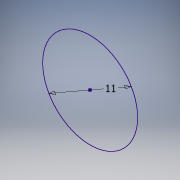
# Autodesk Inventor part: Upper Pneumatic Support
Saved by Autodesk Inventor 2019.4 (Build 234330000, 330)
## iProperties
Created: 2020-01-26
Part Number: Upper Pneumatic Support
Material: Aluminum 6061
Document SubType Name: Modeling
Designer: Mark
Mass: 36.7998 g
Surface Area: 66.9175 cm^2
Volume: 13.6295 cm^3
Density: 2.7 g/cm^3
Appearance: Aluminum - Flat
Author: Mark
Autodesk Inventor part; units mm, degrees
ref_plane "YZ Plane" through (0, 0, 0) normal (1, 0, 0) x (0, 1, 0)
ref_plane "XZ Plane" through (0, 0, 0) normal (0, 1, 0) x (-1, 0, 0)
ref_plane "XY Plane" through (0, 0, 0) normal (0, 0, 1) x (1, 0, 0)
sketch "Sketch1" plane through (0, 0, 0) normal (0, 0, 1) x (1, 0, 0)
  circle A0 centre (0, 0) radius 5.25
  line L0 (-22.5, -22.5) -> (22.5, -22.5)
  line L1 (22.5, -22.5) -> (22.5, 22.5)
  line L2 (22.5, 22.5) -> (-22.5, 22.5)
  line L3 (-22.5, 22.5) -> (-22.5, -22.5)
  line L4 (-22.5, -22.5) -> (22.5, 22.5) construction
  line L5 (22.5, -22.5) -> (-22.5, 22.5) construction
  line L6 (-22.5, 22.5) -> (22.5, 22.5)
  line L7 (22.5, 22.5) -> (22.5, 40)
  line L8 (22.5, 40) -> (-22.5, 40)
  line L9 (-22.5, 40) -> (-22.5, 22.5)
  dimension "d0" = 10.5
  dimension "d1" = 45
  dimension "d2" = 45
  dimension "d3" = 45
  dimension "d4" = 17.5
  constraints: 20 end point, 4 parallel, 2 horizontal, 2 midpoint, 2 perpendicular, 1 centre point, 1 coincident
  measures "d0" diameter of A0
  measures "d1" distance of L2.end L1.end
  measures "d2" distance of L1.end L0.end
  measures "d3" distance of L8.end L7.end
  measures "d4" distance of L7.end L6.end
extrude "Extrusion1" add sketch "Sketch1" along normal blind 5
sketch "Sketch2" plane through (0, 0, 5) normal (0, 0, 1) x (1, 0, 0)
  line L0 (-22.5, 40) -> (-22.5, -22.5) projected
  line L1 (-22.5, 40) -> (22.5, 40)
  line L2 (22.5, 40) -> (22.5, 35)
  line L3 (22.5, 35) -> (-22.5, 35)
  line L4 (-22.5, 35) -> (-22.5, 40)
  point P0 (0, 0)
  dimension "d7" = 45
  dimension "d8" = 5
  constraints: 8 end point, 2 parallel, 1 horizontal, 1 perpendicular
  measures "d7" distance of L2.end L3.end
  measures "d8" distance of L1.end L2.end
extrude "Extrusion2" add sketch "Sketch2" against normal blind 55
sketch "Sketch3" plane through (-22.5, 35, 0) normal (0, -1, 0) x (1, 0, 0)
  line L0 (22.5, -8.25) -> (37.5, -8.25) construction
  line L1 (22.5, -11) -> (37.5, -11)
  line L2 (37.5, -5.5) -> (22.5, -5.5)
  arc A0 (22.5, -5.5) -> (22.5, -11) centre (22.5, -8.25) ccw
  arc A1 (37.5, -11) -> (37.5, -5.5) centre (37.5, -8.25) ccw
  line L3 (22.5, -23.75) -> (37.5, -23.75) construction
  line L4 (22.5, -26.5) -> (37.5, -26.5)
  line L5 (37.5, -21) -> (22.5, -21)
  arc A2 (22.5, -21) -> (22.5, -26.5) centre (22.5, -23.75) ccw
  arc A3 (37.5, -26.5) -> (37.5, -21) centre (37.5, -23.75) ccw
  line L6 (22.5, -23.75) -> (37.5, -23.75) construction
  line L7 (22.5, -39.25) -> (37.5, -39.25) construction
  line L8 (22.5, -42) -> (37.5, -42)
  line L9 (37.5, -36.5) -> (22.5, -36.5)
  arc A4 (22.5, -36.5) -> (22.5, -42) centre (22.5, -39.25) ccw
  arc A5 (37.5, -42) -> (37.5, -36.5) centre (37.5, -39.25) ccw
  line L10 (22.5, -39.25) -> (37.5, -39.25) construction
  line L11 (0, 0) -> (0, -50) projected
  line L12 (45, -50) -> (0, -50) projected
  point P0 (22.5, 0)
  point P1 (30, -8.25)
  point P2 (30, -23.75)
  point P3 (30, -39.25)
  dimension "d11" = 15
  dimension "d12" = 5.5
  dimension "d13" = 15
  dimension "d14" = 0
  dimension "d15" = 5.5
  dimension "d16" = 15
  dimension "d17" = 0
  dimension "d18" = 5.5
  dimension "d19" = 10
  dimension "d20" = 10
  dimension "d21" = 22.5
  dimension "d22" = 22.5
  dimension "d23" = 22.5
  dimension "d24" = 8
  constraints: 28 end point, 12 point on circle, 12 tangent, 6 centre point, 5 parallel, 3 horizontal, 3 midpoint, 2 collinear
  measures "d11" distance of L0.start L0.end
  measures "d12" diameter of A1
  measures "d13" distance of L3.start L3.end
  measures "d14" distance between parallel lines of L3 L6
  measures "d15" diameter of A3
  measures "d16" distance of L7.start L7.end
  measures "d17" distance between parallel lines of L7 L10
  measures "d18" diameter of A5
  measures "d19" distance between parallel lines of L5 L1
  measures "d20" distance between parallel lines of L4 L9
  measures "d21" distance from line of L11 L0.start
  measures "d22" distance from line of L11 L3.start
  measures "d23" distance from line of L11 L7.start
  measures "d24" distance between parallel lines of L12 L8
extrude "Extrusion3" cut sketch "Sketch3" against normal up to next
body "Solid1"
